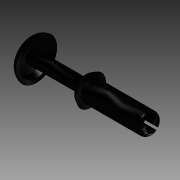
# Autodesk Inventor part: 11-6003
Saved by Autodesk Inventor 2015 SP1 (Build 190203100, 203)
## iProperties
Category: Quick Connect Service Pack
Company: Autodesk Inc.
Created: 2014-11-30
Part Number: 11-6003
Material: Polystyrene, High Impact
Document SubType Name: Modeling
Designer: Matrix
Density: 1.022 g/cm^3
Appearance: Black
Catalog Web Link: http://matrixrobotics.com/
Vendor: Matrix
Author: Autodesk Inc.
Autodesk Inventor part; units mm, degrees
ref_plane "YZ Plane" through (0, 0, 0) normal (1, 0, 0) x (0, 1, 0)
ref_plane "XZ Plane" through (0, 0, 0) normal (0, 1, 0) x (-1, 0, 0)
ref_plane "XY Plane" through (0, 0, 0) normal (0, 0, 1) x (1, 0, 0)
sketch "Sketch1" plane through (0, 0, 0) normal (0, 1, 0) x (-1, 0, 0)
  arc A0 (2.5786, 4.3289) -> (0, 4.6354) centre (0, -6.3646) ccw
  arc A1 (4, 2.8354) -> (2.5786, 4.3289) centre (2.1332, 2.4819) ccw
  line L0 (4, 2.8354) -> (3.2, 2.8354)
  line L1 (3.2, 2.8354) -> (2.8, 3.8354)
  line L2 (2.8, 3.8354) -> (1.225, 3.8354)
  line L3 (1.225, 3.8354) -> (1.225, -7.7996)
  line L4 (1.225, -7.7996) -> (1.275, -7.7996)
  line L5 (1.275, -7.7996) -> (1.275, -6.8996)
  line L6 (1.275, -6.8996) -> (2.3804, -6.8996)
  line L7 (2.3804, -6.8996) -> (2.9, -7.7996)
  line L8 (2.9, -7.7996) -> (1.99, -7.7996)
  line L9 (1.99, -18.7996) -> (1.99, -16.8996)
  line L10 (1.99, -18.7996) -> (1.99, -7.7996)
  spline S0 degree 3 poles (1.99, -18.7996) (1.99, -18.9227) (1.9611, -19.0675) (1.8666, -19.2952) (1.7841, -19.4182) (1.6089, -19.5929) (1.4849, -19.6753) (1.2538, -19.7706) (1.1056, -19.7996) (0.9798, -19.7996) knots 0.751438 0.751438 0.751438 0.751438 0.788362 0.788362 0.82538 0.82538 0.862606 0.862606 0.900353 0.900353 0.900353 0.900353
  line L11 (0.9798, -19.7996) -> (0, -19.7996)
  line L12 (0, 4.6354) -> (0, -19.7996)
  point P0 (0, 0)
  point P1 (0, 0)
  constraints: 26 end point, 4 point on circle, 2 centre point, 1 vertical, 2 other
revolve "Revolution1" add sketch "Sketch1" angle 360 about axis through (0, 0, 4.6354) along (0, 0, -1)
sketch "Sketch2" plane through (0, 0, -19.7996) normal (0, 0, -1) x (-1, 0, 0)
  line L0 (0, 0.2829) -> (-1.2657, 1.5485)
  arc A0 (0.5514, 0.8343) -> (-0.5514, 0.8343) centre (0, 0) ccw
  line L1 (1.2657, 1.5485) -> (0, 0.2829)
  line L2 (0, -0.2829) -> (1.2656, -1.5485)
  arc A1 (-0.5514, -0.8343) -> (0.5514, -0.8343) centre (0, 0) ccw
  line L3 (-1.2657, -1.5485) -> (0, -0.2829)
  line L4 (0.2829, 0) -> (1.5485, 1.2657)
  arc A2 (0.8343, -0.5514) -> (0.8343, 0.5514) centre (0, 0) ccw
  line L5 (1.5485, -1.2656) -> (0.2829, 0)
  arc A3 (-0.8343, 0.5514) -> (-0.8343, -0.5514) centre (0, 0) ccw
  line L6 (-0.2829, 0) -> (-1.5485, -1.2656)
  line L7 (-1.5485, 1.2657) -> (-0.2829, 0)
  arc A4 (1.2657, 1.5485) -> (-1.2657, 1.5485) centre (0, 0) ccw
  circle A5 centre (0, 0) radius 2
  point P0 (0, 0)
  point P1 (0, 0)
  constraints: 16 end point, 10 point on circle, 8 point on line, 5 centre point, 1 coincident, 11 other
extrude "Extrusion1" cut sketch "Sketch2" against normal blind 3 contours L1 A5 L4 L5 L2 L3 L6 L7 L0
body "Solid1"
